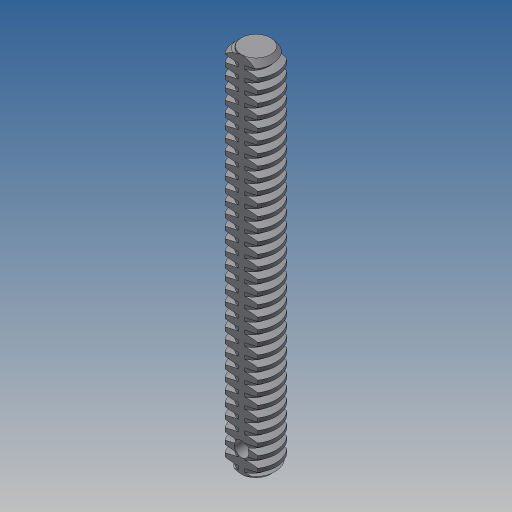
# Autodesk Inventor part: Vis
Saved by Autodesk Inventor 2024.1 (Build 281209000, 209)
## iProperties
Created: 2023-10-23
Part Number: Vis
Project: Nom Projet
Material: .
Description: Nom pièce
Document SubType Name: Modeling
Designer: Jean-Marc Vulliamy
Authority: brut Ø
Mass: 0.00696289 g
Surface Area: 50.5334 cm^2
Volume: 6.96289 cm^3
Density: 0.001 g/cm^3
Appearance: Par défaut
Material number: ---
Author: Jean-Marc Vulliamy
Autodesk Inventor part; units mm, degrees
ref_plane "Plan YZ" through (0, 0, 0) normal (1, 0, 0) x (0, 1, 0)
ref_plane "Plan XZ" through (0, 0, 0) normal (0, 1, 0) x (-1, 0, 0)
ref_plane "Plan XY" through (0, 0, 0) normal (0, 0, 1) x (1, 0, 0)
sketch "Esquisse1" plane through (0, 0, 0) normal (0, 0, 1) x (1, 0, 0)
  circle A0 centre (0, 0) radius 6
  dimension "d0" = 12
  constraints: 1 centre point, 1 coincident
  measures "d0" diameter of A0
extrude "Extrusion1" add sketch "Esquisse1" along normal blind 100
chamfer "Chanfrein1" distance 2 angle 45 2 edges at (-6, 0, 100) (-6, 0, 0)
sketch "Esquisse6" plane through (0, 0, 0) normal (0, 1, 0) x (-1, 0, 0)
  line L0 (-6, 0) -> (-6, 100) construction
  line L1 (-11.4533, 0) -> (1.9089, 0) construction
  line L2 (-7.899, 0.5088) -> (-2.301, -0.9912) construction
  line L3 (-2.301, -0.9912) -> (-7.899, -2.4912) construction
  line L4 (-2.301, -0.9912) -> (-9.5444, -0.9912) construction
  line L5 (0, -31.3269) -> (0, 121.8878) construction
  line L6 (-7.899, 0.5088) -> (-7.899, -2.4912) construction
  line L7 (-5.1, 4.2722) -> (-5.1, -9.8902) construction
  line L8 (-2.301, -0.9912) -> (-2.301, -2.3746) construction
  line L9 (-4.1, 0) -> (-4.1, -4.3642) construction
  line L10 (-6, -1.9823) -> (-4.1, -1.4732)
  line L11 (-4.1, -1.4732) -> (-4.1, -0.5091)
  line L12 (-4.1, -0.5091) -> (-6, 0)
  line L13 (-6, 0) -> (-6, -1.9823)
  point P0 (0, 0)
  dimension "d5" = 30
  dimension "d6" = 3
  dimension "d8" = 10.2
  dimension "d11" = 1.9
  constraints: 22 end point, 7 point on line, 4 vertical, 1 coincident, 1 collinear, 1 horizontal, 1 parallel, 1 vertical alignment, 2 other
  measures "d5" angle of L3 L2
  measures "d6" distance of L2.start L3.end
  measures "d8" diameter of L7 L5
  measures "d11" distance between parallel lines of L9 L0
coil "Hélicoïde1" sketch "Esquisse6" operation cut axis through (0, 0, 0) along (0, 0, 1) pitch 3 turns 34.333333 hand right
sketch "Esquisse7" plane through (0, 0, 0) normal (0, 0, 1) x (1, 0, 0)
  line L0 (6, 4) -> (-6, 4)
  line L1 (-6, 4) -> (-6, -4)
  line L2 (-6, -4) -> (6, -4)
  line L3 (6, -4) -> (6, 4)
  line L4 (0, 8.4) -> (0, -8.4) construction
  line L5 (-8.4, 0) -> (8.4, 0) construction
  circle A0 centre (0, 0) radius 6 construction
  arc A1 (4.4721, 4) -> (-4.4721, 4) centre (0, 0) ccw
  arc A2 (-4.4721, -4) -> (4.4721, -4) centre (0, 0) ccw
  dimension "d20" = 8
  constraints: 8 end point, 8 point on circle, 4 point on line, 2 centre point, 2 concentric, 2 parallel, 2 tangent, 1 horizontal, 1 perpendicular, 1 other
  measures "d20" distance between parallel lines of L2 L0
extrude "Extrusion2" cut sketch "Esquisse7" along normal through all contours L0 A1 | A2 L2
sketch "Esquisse9" plane through (2.6893, -4, 2.2347) normal (0, -1, 0) x (0.985457, 0, 0.1699249)
  line L0 (17.361, 116.5096) -> (-6.4285, -21.4544) construction
  point P0 (-3.03, -1.7452)
  point P1 (-2.0104, 4.1675)
  dimension "d36" = 6
  constraints: 1 point on line
  measures "d36" distance of point (-3.03, -1.745) point (-2.01, 4.167)
hole "Perçage2" at (0, -4, 6) direction (0, 1, 0) diameter 4 end through all
equation "\"d0\" = Dnominal"
equation "\"d6\" = Pas"
equation "\"d8\" = Dnominal - 0.6 * Pas"
equation "\"d11\" = 0.5 * Pas + Jeu"
equation "\"d12\" = d6"
equation "\"Pas\" = 3"
equation "\"Jeu\" = 0.4"
equation "\"Dnominal\" = 12"
